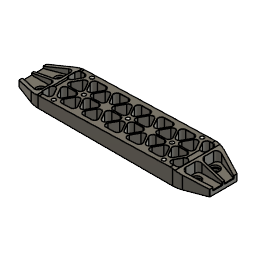
BUBBLED (Autodesk Fusion 360 design; units mm, degrees)
part number: 2026-08-30-08-59-27-515
Autodesk Fusion 360 part; units mm, degrees
note: some values were not read from the file. Chosen so that the rebuilt part matches the saved one: which face or edge a step refers to; how an offset face is resized.
sketch "Sketch1" plane through (0, 0, 0) normal (0, 1, 0) x (1, 0, 0)
  line L0 (30.0059, 0) -> (173.1941, 0)
  line L1 (203.2, -9.789) -> (203.2, -38.471)
  line L2 (173.1941, -48.26) -> (30.0059, -48.26)
  line L3 (0, -38.471) -> (0, -9.789)
  line L4 (0.2472, -9.4323) -> (21.0874, -1.6172)
  line L5 (21.0874, -46.6428) -> (0.2472, -38.8277)
  line L6 (182.1126, -1.6172) -> (202.9528, -9.4323)
  line L7 (202.9528, -38.8277) -> (182.1126, -46.6428)
  arc A0 (21.0874, -46.6428) -> (30.0059, -48.26) centre (30.0059, -22.86) ccw
  arc A1 (173.1941, -48.26) -> (182.1126, -46.6428) centre (173.1941, -22.86) ccw
  arc A2 (182.1126, -1.6172) -> (173.1941, 0) centre (173.1941, -25.4) ccw
  arc A3 (30.0059, 0) -> (21.0874, -1.6172) centre (30.0059, -25.4) ccw
  arc A4 (0.2472, -9.4323) -> (0, -9.789) centre (0.381, -9.789) ccw
  arc A5 (0, -38.471) -> (0.2472, -38.8277) centre (0.381, -38.471) ccw
  arc A6 (202.9528, -38.8277) -> (203.2, -38.471) centre (202.819, -38.471) ccw
  arc A7 (203.2, -9.789) -> (202.9528, -9.4323) centre (202.819, -9.789) ccw
  point P0 (0, -9.525)
  point P1 (25.4, 0)
  dimension "d5" = 25.4
  dimension "d6" = 9.525
  dimension "d13" = 25.4
  dimension "d14" = 0.381
  constraint horizontal L0
  constraint vertical L1
  constraint horizontal L2
  constraint vertical L3
  constraint tangent L5 A0
  constraint tangent L2 A0
  constraint tangent L7 A1
  constraint tangent L2 A1
  constraint equal A0 A1
  constraint tangent L6 A2
  constraint tangent L0 A2
  constraint equal A0 A2
  constraint coincident P1 L4
  constraint coincident L0 P1
  constraint tangent L4 A3
  constraint tangent L0 A3
  constraint equal A0 A3
  constraint coincident P0 L4
  constraint coincident L3 P0
  constraint tangent L4 A4
  constraint tangent L3 A4
  constraint tangent L5 A5
  constraint tangent L3 A5
  constraint equal A4 A5
  constraint tangent L7 A6
  constraint tangent L1 A6
  constraint equal A4 A6
  constraint tangent L6 A7
  constraint tangent L1 A7
  constraint equal A4 A7
  measures "d5" distance of origin P1
  measures "d6" distance of origin P0
  measures "d13" radius of A0
  measures "d14" radius of A4
extrude "Extrude1" add sketch "Sketch1" along normal blind 22.2504
sketch "Sketch2" plane through (0, 0, 0) normal (0, -1, 0) x (1, 0, 0)
  arc A0 (203.2, 38.471) -> (202.9528, 38.8277) centre (202.819, 38.471) ccw
  line L0 (202.9528, 38.8277) -> (182.1126, 46.6428)
  arc A1 (182.1126, 46.6428) -> (173.1941, 48.26) centre (173.1941, 22.86) ccw
  line L1 (173.1941, 48.26) -> (30.0059, 48.26)
  arc A2 (30.0059, 48.26) -> (21.0874, 46.6428) centre (30.0059, 22.86) ccw
  line L2 (21.0874, 46.6428) -> (0.2472, 38.8277)
  arc A3 (0.2472, 38.8277) -> (0, 38.471) centre (0.381, 38.471) ccw
  line L3 (0, 38.471) -> (0, 9.789)
  arc A4 (0, 9.789) -> (0.2472, 9.4323) centre (0.381, 9.789) ccw
  line L4 (0.2472, 9.4323) -> (21.0874, 1.6172)
  arc A5 (21.0874, 1.6172) -> (30.0059, 0) centre (30.0059, 25.4) ccw
  line L5 (30.0059, 0) -> (173.1941, 0)
  arc A6 (173.1941, 0) -> (182.1126, 1.6172) centre (173.1941, 25.4) ccw
  line L6 (182.1126, 1.6172) -> (202.9528, 9.4323)
  arc A7 (202.9528, 9.4323) -> (203.2, 9.789) centre (202.819, 9.789) ccw
  line L7 (203.2, 9.789) -> (203.2, 38.471)
  circle A8 centre (101.6, 24.13) radius 3.4925
  circle A9 centre (54.6608, 24.13) radius 3.4925
  circle A10 centre (148.5392, 24.13) radius 3.4925
  dimension "d17" = 6.985
  dimension "d18" = 24.13
  dimension "d19" = 101.6
  dimension "d22" = 46.9392
  dimension "d23" = 0
  measures "d17" diameter of A8
  measures "d18" distance of L1 A8.centre
  measures "d19" distance of L3 A8.centre
extrude "Extrude2" cut sketch "Sketch2" against normal blind 5.08
sketch "Sketch3" plane through (0, 22.2504, 0) normal (0, 1, 0) x (-1, 0, 0)
  arc A0 (-202.9528, 38.8277) -> (-203.2, 38.471) centre (-202.819, 38.471) ccw
  line L0 (-203.2, 38.471) -> (-203.2, 9.789)
  arc A1 (-203.2, 9.789) -> (-202.9528, 9.4323) centre (-202.819, 9.789) ccw
  line L1 (-202.9528, 9.4323) -> (-182.1126, 1.6172)
  arc A2 (-182.1126, 1.6172) -> (-173.1941, 0) centre (-173.1941, 25.4) ccw
  line L2 (-173.1941, 0) -> (-30.0059, 0)
  arc A3 (-30.0059, 0) -> (-21.0874, 1.6172) centre (-30.0059, 25.4) ccw
  line L3 (-21.0874, 1.6172) -> (-0.2472, 9.4323)
  arc A4 (-0.2472, 9.4323) -> (0, 9.789) centre (-0.381, 9.789) ccw
  line L4 (0, 9.789) -> (0, 38.471)
  arc A5 (0, 38.471) -> (-0.2472, 38.8277) centre (-0.381, 38.471) ccw
  line L5 (-0.2472, 38.8277) -> (-21.0874, 46.6428)
  arc A6 (-21.0874, 46.6428) -> (-30.0059, 48.26) centre (-30.0059, 22.86) ccw
  line L6 (-30.0059, 48.26) -> (-173.1941, 48.26)
  arc A7 (-173.1941, 48.26) -> (-182.1126, 46.6428) centre (-173.1941, 22.86) ccw
  line L7 (-182.1126, 46.6428) -> (-202.9528, 38.8277)
  line L8 (-101.6, -25.4) -> (-101.6, 76.2) construction
  point P0 (-101.6, 24.13)
  point P1 (-42.9514, 3.81)
  point P2 (-42.9514, 44.45)
  point P3 (-54.6608, 24.13)
  point P4 (-148.5392, 24.13)
  point P5 (-160.2486, 3.81)
  point P6 (-160.2486, 44.45)
  dimension "d26" = 24.13
  dimension "d27" = 101.6
  dimension "d28" = 3.81
  dimension "d29" = 42.9514
  dimension "d30" = 42.9514
  dimension "d31" = 44.45
  dimension "d32" = 24.13
  dimension "d33" = 54.6608
  constraint vertical L8
  constraint symmetric L8 P1 P5
  constraint symmetric L8 P2 P6
  constraint symmetric L8 P3 P4
  measures "d26" distance of L2 P0
  measures "d27" distance of L4 P0
  measures "d28" distance of L2 P1
  measures "d29" distance of L4 P1
  measures "d30" distance of L4 P2
  measures "d31" distance of L2 P2
  measures "d32" distance of L2 P3
  measures "d33" distance of L4 P3
sketch "Sketch4" plane through (0, 22.2504, 0) normal (0, 1, 0) x (-1, 0, 0)
  line L0 (-27.94, 7.0358) -> (-27.94, 13.7682)
  line L1 (-33.9594, 15.3811) -> (-37.8464, 8.6487)
  line L2 (-35.0528, 3.81) -> (-31.1658, 3.81)
  line L3 (-173.1941, 0) -> (-30.0059, 0)
  line L4 (0, 9.789) -> (0, 38.471)
  arc A0 (-31.1658, 3.81) -> (-27.94, 7.0358) centre (-31.1658, 7.0358) ccw
  arc A1 (-37.8464, 8.6487) -> (-35.0528, 3.81) centre (-35.0528, 7.0358) ccw
  arc A2 (-27.94, 13.7682) -> (-33.9594, 15.3811) centre (-31.1658, 13.7682) ccw
  line L5 (-101.6, -25.4) -> (-101.6, 76.2) construction
  line L6 (-169.2406, 15.3811) -> (-165.3536, 8.6487)
  arc A3 (-169.2406, 15.3811) -> (-175.26, 13.7682) centre (-172.0342, 13.7682) ccw
  arc A4 (-168.1473, 3.81) -> (-165.3536, 8.6487) centre (-168.1473, 7.0358) ccw
  line L7 (-168.1473, 3.81) -> (-172.0342, 3.81)
  arc A5 (-175.26, 7.0358) -> (-172.0342, 3.81) centre (-172.0342, 7.0358) ccw
  line L8 (-175.26, 7.0358) -> (-175.26, 13.7682)
  dimension "d34" = 3.81
  dimension "d35" = 27.94
  dimension "d36" = 60
  dimension "d37" = 3.2258
  dimension "d102" = 101.6
  constraint vertical L0
  constraint perpendicular L0 L2
  constraint tangent L0 A0
  constraint tangent L2 A0
  constraint tangent L1 A1
  constraint tangent L2 A1
  constraint equal A0 A1
  constraint tangent L0 A2
  constraint tangent L1 A2
  constraint equal A0 A2
  constraint perpendicular L3 L5
  constraint symmetric L0.start L5 A5.start
  constraint symmetric L2.end L5 L7.end
  constraint symmetric A0 L5 A5
  constraint symmetric L1.end L5 L6.end
  constraint symmetric L2.start L5 A4.start
  constraint symmetric A1 L5 A4
  constraint symmetric L0.end L5 A3.end
  constraint symmetric L1.start L5 L6.start
  constraint symmetric A2 L5 A3
  measures "d34" distance of L2 L3
  measures "d35" distance of L0 L4
  measures "d36" angle of L1 L2
  measures "d37" radius of A0
  measures "d102" distance of origin L5
sketch "Sketch5" plane through (0, 22.2504, 0) normal (0, 1, 0) x (-1, 0, 0)
  line L0 (-42.929, 3.81) -> (-31.1973, 24.13) construction
  line L1 (-31.1973, 24.13) -> (-42.929, 44.45) construction
  line L2 (-42.929, 44.45) -> (-66.3926, 44.45) construction
  line L3 (-66.3926, 44.45) -> (-78.1243, 24.13) construction
  line L4 (-78.1243, 24.13) -> (-66.3926, 3.81) construction
  line L5 (-66.3926, 3.81) -> (-42.929, 3.81) construction
  line L6 (-54.6608, 24.13) -> (-78.1243, 24.13) construction
  line L7 (-66.0614, 3.81) -> (-66.3926, 44.45) construction
  line L8 (-63.3332, 10.1409) -> (-58.7834, 18.0213)
  line L9 (-61.577, 22.86) -> (-70.6783, 22.86)
  line L10 (-73.4716, 18.0208) -> (-68.9202, 10.1404)
  line L11 (-173.1941, 0) -> (-30.0059, 0) construction
  arc A0 (-68.9202, 10.1404) -> (-63.3332, 10.1409) centre (-66.1268, 11.7538) ccw
  arc A1 (-58.7834, 18.0213) -> (-61.577, 22.86) centre (-61.577, 19.6342) ccw
  arc A2 (-70.6783, 22.86) -> (-73.4716, 18.0208) centre (-70.6783, 19.6342) ccw
  line L12 (-58.7755, 4.7847) -> (-49.6751, 4.7862)
  arc A3 (-61.5697, 9.6234) -> (-58.7755, 4.7847) centre (-58.7761, 8.0105) ccw
  line L13 (-57.0191, 17.5054) -> (-61.5697, 9.6234)
  arc A4 (-49.6751, 4.7862) -> (-46.882, 9.6249) centre (-49.6757, 8.012) ccw
  arc A5 (-51.4318, 17.5054) -> (-57.0191, 17.5054) centre (-54.2254, 15.8925) ccw
  line L14 (-46.882, 9.6249) -> (-51.4318, 17.5054)
  line L15 (-39.9647, 10.8939) -> (-35.4158, 18.7758)
  arc A6 (-45.5522, 10.8934) -> (-39.9647, 10.8939) centre (-42.7586, 12.5063) ccw
  line L16 (-50.1028, 18.7754) -> (-45.5522, 10.8934)
  arc A7 (-35.4158, 18.7758) -> (-38.2097, 23.6141) centre (-38.2097, 20.3883) ccw
  arc A8 (-47.3092, 23.6141) -> (-50.1028, 18.7754) centre (-47.3092, 20.3883) ccw
  line L17 (-38.2097, 23.6141) -> (-47.3092, 23.6141)
  line L18 (-35.85, 30.2392) -> (-40.4014, 38.1196)
  arc A9 (-38.6433, 25.4) -> (-35.85, 30.2392) centre (-38.6433, 28.6258) ccw
  line L19 (-47.7446, 25.4) -> (-38.6433, 25.4)
  arc A10 (-40.4014, 38.1196) -> (-45.9884, 38.1191) centre (-43.1948, 36.5062) ccw
  arc A11 (-50.5382, 30.2387) -> (-47.7446, 25.4) centre (-47.7446, 28.6258) ccw
  line L20 (-45.9884, 38.1191) -> (-50.5382, 30.2387)
  line L21 (-50.5461, 43.4753) -> (-59.6465, 43.4738)
  arc A12 (-47.7519, 38.6366) -> (-50.5461, 43.4753) centre (-50.5455, 40.2495) ccw
  line L22 (-52.3025, 30.7546) -> (-47.7519, 38.6366)
  arc A13 (-59.6465, 43.4738) -> (-62.4396, 38.6351) centre (-59.6459, 40.248) ccw
  arc A14 (-57.8898, 30.7546) -> (-52.3025, 30.7546) centre (-55.0962, 32.3675) ccw
  line L23 (-62.4396, 38.6351) -> (-57.8898, 30.7546)
  line L24 (-69.3569, 37.3661) -> (-73.9058, 29.4842)
  arc A15 (-63.7694, 37.3666) -> (-69.3569, 37.3661) centre (-66.563, 35.7537) ccw
  line L25 (-59.2188, 29.4846) -> (-63.7694, 37.3666)
  arc A16 (-73.9058, 29.4842) -> (-71.1119, 24.6459) centre (-71.1119, 27.8717) ccw
  arc A17 (-62.0124, 24.6459) -> (-59.2188, 29.4846) centre (-62.0124, 27.8717) ccw
  line L26 (-71.1119, 24.6459) -> (-62.0124, 24.6459)
  point P0 (-54.6608, 24.13)
  point P1 (-54.6608, 24.13)
  dimension "d38" = 20.32
  dimension "d39" = 1.27
  dimension "d40" = 59.991
  dimension "d41" = 3.2258
  dimension "d43" = 360
  constraint coincident P0 L6.start
  constraint coincident L5 L7.start
  constraint horizontal L6
  constraint parallel L6 L9
  constraint tangent L8 A0
  constraint tangent L10 A0
  constraint tangent L8 A1
  constraint tangent L9 A1
  constraint equal A0 A1
  constraint tangent L9 A2
  constraint tangent L10 A2
  constraint equal A0 A2
  measures "d38" distance of P1 L5
  measures "d39" distance of L6 L9
  measures "d40" angle of L10 L11
  measures "d41" radius of A0
sketch "Sketch6" plane through (0, 22.2504, 0) normal (0, 1, 0) x (-1, 0, 0)
  line L0 (-57.0191, 17.5054) -> (-61.5697, 9.6234) construction
  arc A0 (-61.5697, 9.6234) -> (-58.7755, 4.7847) centre (-58.7761, 8.0105) ccw construction
  line L1 (-58.7755, 4.7847) -> (-49.6751, 4.7862) construction
  arc A1 (-49.6751, 4.7862) -> (-46.882, 9.6249) centre (-49.6757, 8.012) ccw construction
  line L2 (-46.882, 9.6249) -> (-51.4318, 17.5054) construction
  arc A2 (-51.4318, 17.5054) -> (-57.0191, 17.5054) centre (-54.2254, 15.8925) ccw construction
  line L3 (-66.0614, 3.81) -> (-66.3926, 44.45)
  arc A3 (-73.3622, 4.6659) -> (-70.6472, 9.5495) centre (-73.4142, 7.8913) ccw
  line L4 (-73.3622, 4.6659) -> (-82.4614, 4.5191)
  arc A4 (-85.333, 9.3116) -> (-82.4614, 4.5191) centre (-82.5134, 7.7444) ccw
  line L5 (-85.333, 9.3116) -> (-80.9122, 17.2651)
  arc A5 (-75.3257, 17.3562) -> (-80.9122, 17.2651) centre (-78.0927, 15.698) ccw
  line L6 (-75.3257, 17.3562) -> (-70.6472, 9.5495)
  line L7 (-101.6, -25.4) -> (-101.6, 72.1933) construction
  arc A6 (-120.7386, 4.5191) -> (-117.867, 9.3116) centre (-120.6866, 7.7444) ccw
  line L8 (-117.867, 9.3116) -> (-122.2878, 17.2651)
  line L9 (-127.8743, 17.3562) -> (-132.5528, 9.5495)
  arc A7 (-132.5528, 9.5495) -> (-129.8378, 4.6659) centre (-129.7858, 7.8913) ccw
  arc A8 (-122.2878, 17.2651) -> (-127.8743, 17.3562) centre (-125.1073, 15.698) ccw
  line L10 (-129.8378, 4.6659) -> (-120.7386, 4.5191)
  dimension "d95" = 101.6
  constraint symmetric L0.start L3 A5.start
  constraint symmetric L0.end L3 A3.end
  constraint symmetric A0.end L3 A3.start
  constraint symmetric A0 L3 A3
  constraint symmetric L1.end L3 L4.end
  constraint symmetric A1.end L3 A4.start
  constraint symmetric A1 L3 A4
  constraint symmetric L2.end L3 L5.end
  constraint symmetric A2 L3 A5
  constraint vertical L7
  constraint symmetric A3.end L7 L9.end
  constraint symmetric A3.start L7 A7.end
  constraint symmetric A3 L7 A7
  constraint symmetric L4.end L7 A6.start
  constraint symmetric A4.start L7 A6.end
  constraint symmetric A4 L7 A6
  constraint symmetric L5.end L7 L8.end
  constraint symmetric A5.start L7 L9.start
  constraint symmetric A5 L7 A8
  measures "d95" distance of origin L7
sketch "Sketch7" plane through (0, 22.2504, 0) normal (0, 1, 0) x (-1, 0, 0)
  line L0 (0, 9.789) -> (0, 38.471)
  line L1 (-173.1941, 0) -> (-30.0059, 0)
  line L2 (-101.6, -25.4) -> (-101.6, 76.2)
  point P0 (-18.923, 14.1732)
  point P1 (-18.923, 34.0868)
  point P2 (-184.277, 14.1732)
  point P3 (-184.277, 34.0868)
  dimension "d45" = 18.923
  dimension "d46" = 18.923
  dimension "d47" = 14.1732
  dimension "d48" = 34.0868
  constraint symmetric P0 L2 P2
  constraint symmetric P1 L2 P3
  measures "d45" distance of P0 L0
  measures "d46" distance of P1 L0
  measures "d47" distance of P0 L1
  measures "d48" distance of P1 L1
sketch "Sketch8" plane through (0, 22.2504, 0) normal (0, 1, 0) x (-1, 0, 0)
  line L0 (12.6994, 18.0851) -> (12.6994, 22.86)
  line L1 (12.6994, 22.86) -> (-21.59, 22.86)
  line L2 (-25.4, 19.05) -> (-25.4, 9.2956)
  line L3 (-20.2522, 5.7282) -> (12.6994, 18.0851)
  line L4 (-21.0874, 1.6172) -> (-0.2472, 9.4323)
  line L5 (0, 9.789) -> (0, 38.471)
  line L6 (-173.1941, 0) -> (-30.0059, 0)
  line L7 (12.7, 24.13) -> (-76.2, 24.13) construction
  arc A0 (-25.4, 9.2956) -> (-20.2522, 5.7282) centre (-21.59, 9.2956) ccw
  arc A1 (-21.59, 22.86) -> (-25.4, 19.05) centre (-21.59, 19.05) ccw
  line L8 (12.6994, 25.4) -> (-21.59, 25.4)
  arc A2 (-25.4, 29.21) -> (-21.59, 25.4) centre (-21.59, 29.21) ccw
  line L9 (-25.4, 29.21) -> (-25.4, 38.9644)
  arc A3 (-20.2522, 42.5318) -> (-25.4, 38.9644) centre (-21.59, 38.9644) ccw
  line L10 (-20.2522, 42.5318) -> (12.6994, 30.1749)
  line L11 (12.6994, 30.1749) -> (12.6994, 25.4)
  line L12 (-101.6, -25.4) -> (-101.6, 76.2) construction
  line L13 (-177.8, 19.05) -> (-177.8, 9.2956)
  arc A4 (-182.9478, 5.7282) -> (-177.8, 9.2956) centre (-181.61, 9.2956) ccw
  line L14 (-182.9478, 5.7282) -> (-215.8994, 18.0851)
  line L15 (-215.8994, 18.0851) -> (-215.8994, 22.86)
  line L16 (-215.8994, 22.86) -> (-181.61, 22.86)
  arc A5 (-177.8, 19.05) -> (-181.61, 22.86) centre (-181.61, 19.05) ccw
  arc A6 (-181.61, 25.4) -> (-177.8, 29.21) centre (-181.61, 29.21) ccw
  line L17 (-215.8994, 25.4) -> (-181.61, 25.4)
  line L18 (-177.8, 29.21) -> (-177.8, 38.9644)
  arc A7 (-177.8, 38.9644) -> (-182.9478, 42.5318) centre (-181.61, 38.9644) ccw
  line L19 (-182.9478, 42.5318) -> (-215.8994, 30.1749)
  line L20 (-215.8994, 30.1749) -> (-215.8994, 25.4)
  dimension "d50" = 3.556
  dimension "d51" = 25.4
  dimension "d52" = 22.86
  dimension "d53" = 3.81
  dimension "d54" = 24.13
  constraint vertical L0
  constraint perpendicular L0 L1
  constraint perpendicular L1 L2
  constraint parallel L3 L4
  constraint horizontal L7
  constraint tangent L2 A0
  constraint tangent L3 A0
  constraint tangent L1 A1
  constraint tangent L2 A1
  constraint equal A0 A1
  constraint symmetric L0.start L7 L10.end
  constraint symmetric L0.end L7 L8.start
  constraint symmetric L7 L2.end L9.end
  constraint symmetric L7 L3.start A3.start
  constraint symmetric L7 A0 A3
  constraint symmetric L7 L1.end L8.end
  constraint symmetric L7 L2.start A2.start
  constraint symmetric L7 A1 A2
  constraint symmetric L0.start L12 L14.end
  constraint symmetric L0.end L12 L15.end
  constraint symmetric L2.end L12 L13.end
  constraint symmetric L3.start L12 A4.start
  constraint symmetric A0 L12 A4
  constraint symmetric L1.end L12 L16.end
  constraint symmetric L2.start L12 L13.start
  constraint symmetric A1 L12 A5
  constraint symmetric L8.start L12 L17.start
  constraint symmetric L8.end L12 A6.start
  constraint symmetric A2.start L12 A6.end
  constraint symmetric A2 L12 A6
  constraint symmetric L9.end L12 L18.end
  constraint symmetric A3.start L12 A7.end
  constraint symmetric A3 L12 A7
  constraint symmetric L10.end L12 L19.end
  measures "d50" distance of L3 L4
  measures "d51" distance of L2 L5
  measures "d52" distance of L1 L6
  measures "d53" radius of A0
  measures "d54" distance of L6 L7
sketch "Sketch9" plane through (0, 0, 48.26) normal (0, 0, 1) x (1, 0, 0)
  line L0 (30.0059, 5.08) -> (173.1941, 5.08) construction
  line L1 (173.1941, 5.08) -> (173.1941, 22.2504)
  line L2 (173.1941, 22.2504) -> (30.0059, 22.2504)
  line L3 (30.0059, 22.2504) -> (30.0059, 5.08)
  line L4 (30.0059, 5.08) -> (173.1941, 5.08)
  line L5 (0, 5.08) -> (0, 11.4554)
  line L6 (30.0059, 5.08) -> (30.0059, 17.1704)
  line L7 (0, 11.4554) -> (30.0059, 17.1704)
  line L8 (30.0059, 22.2504) -> (0, 22.2504)
  line L9 (0, 22.2504) -> (0, 11.4554)
  line L10 (30.0059, 17.1704) -> (30.0059, 22.2504)
  line L11 (30.0059, 22.2504) -> (203.2, 22.2504)
  line L12 (203.2, 22.2504) -> (203.2, 12.0904)
  line L13 (30.0059, 17.1704) -> (173.1941, 21.4376)
  line L14 (203.2, 12.0904) -> (173.1941, 21.4376)
  point P0 (0, 5.08)
  dimension "d57" = 10.795
  dimension "d58" = 5.08
  dimension "d61" = 10.16
  dimension "d62" = 21.4376
  constraint coincident P0 L5.start
  constraint vertical L5
  constraint coincident L0.start L3.end
  constraint coincident L3 L6.end
  constraint coincident L2.end L3.start
  constraint perpendicular L3 L8
  constraint perpendicular L8 L9
  constraint perpendicular L3 L11
  constraint perpendicular L11 L12
  constraint coincident L1 L13.end
  measures "d57" distance of L2 L5.end
  measures "d58" distance of L2 L6.end
  measures "d61" distance of L11.end L12.end
  measures "d62" vertical distance of origin L13.end
extrude "Extrude3" cut sketch "Sketch9" against normal blind 76.2 contours L1 L2 L3 L10 L11 L13 | L1 L11 L12 L14 | L3 L7 L8 L9 L10
fillet "Fillet1" radius 15.24 2 edges at (173.1941, 21.4376, 24.13) (30.0059, 17.1704, 24.13)
hole "Hole1" at (42.9514, 22.2504, 3.81) at (54.6608, 22.2504, 24.13) at (42.9514, 22.2504, 44.45) at (160.2486, 22.2504, 44.45) at (148.5392, 22.2504, 24.13) at (160.2486, 22.2504, 3.81) at (101.6, 22.2504, 24.13) direction (0, -1, 0) diameter 3.9688 depth 22.8203 tip angle 118
thread "Thread1" "ANSI Unified Screw Threads 0.19(#10) 10-32 UNF 10-32 UNF 2B" major diameter 4.826 minor diameter 4.064 pitch 0.7937 angle 60 resizes the face on face at (44.846, 9.2575, 4.4001) on face at (162.1424, 10.4227, 4.4025) on face at (56.6452, 5.9881, 24.1326) on face at (44.846, 9.2575, 45.0401) on face at (162.1424, 10.4227, 45.0425) on face at (103.5603, 6.4541, 24.4383) on face at (150.4364, 6.9198, 24.7116)
extrude "Extrude4" cut sketch "Sketch8" against normal blind 12.7 contours L1 L2 L3 L5 A0 A1 | L5 L8 A2 L9 A3 L10 | L13 A4 L14 L15 L16 A5 | A6 L17 L18 A7 L19 L20
fillet "Fillet2" radius 0.381 12 edges at (203.2, 10.8204, 13.3228) (203.2, 9.5504, 18.0914) (203.2, 10.8204, 22.86) (203.2, 10.8204, 25.4) (203.2, 9.5504, 30.1686) (203.2, 10.8204, 34.9372) (0, 10.5029, 13.3228) (0, 9.5504, 18.0914) (0, 10.5029, 22.86) (0, 10.5029, 25.4) (0, 9.5504, 30.1686) (0, 10.5029, 34.9372)
sketch "Sketch10" plane through (0, 9.5504, 0) normal (0, 1, 0) x (-1, 0, 0)
  line L0 (-0.381, 25.4) -> (-0.381, 35.106)
  arc A0 (-0.5148, 35.1302) -> (-0.381, 35.106) centre (-0.381, 35.487) ccw
  line L1 (-0.5148, 35.1302) -> (-20.2522, 42.5318)
  arc A1 (-20.2522, 42.5318) -> (-25.4, 38.9644) centre (-21.59, 38.9644) ccw
  line L2 (-25.4, 38.9644) -> (-25.4, 29.21)
  arc A2 (-25.4, 29.21) -> (-21.59, 25.4) centre (-21.59, 29.21) ccw
  line L3 (-21.59, 25.4) -> (-0.381, 25.4)
  line L4 (0, 9.789) -> (0, 38.471)
  point P0 (-184.277, 34.0868)
  point P1 (-184.277, 14.1732)
  point P2 (-18.923, 14.1732)
  point P3 (-18.923, 34.0868)
  dimension "d86" = 18.8516
hole "Hole3" at (18.923, 9.5504, 34.0868) at (18.923, 9.5504, 14.1732) at (184.277, 9.5504, 14.1732) at (184.277, 9.5504, 34.0868) direction (0, -1, 0) diameter 6.604 depth 5.08 tip angle 118 counterbore diameter 9.652 counterbore depth 2.032
extrude "Extrude5" cut sketch "Sketch5" against normal blind 20.2406
pattern_linear "R-Pattern1" count 3 spacing 47.0297 along (0.999556, 0.029788, 0) of "Extrude5"
extrude "Extrude6" cut sketch "Sketch6" against normal blind 20.2406
ref_plane "WorkPlane1" through (0, 0, 24.13) normal (0, 0, 1) x (1, 0, 0)
mirror "Mirror1" about plane through (0, 0, 24.13) normal (0, 0, 1) of "Extrude6"
extrude "Extrude7" cut sketch "Sketch4" against normal blind 20.2406
mirror "Mirror2" about plane through (0, 0, 24.13) normal (0, 0, 1) of "Extrude7"
chamfer "Chamfer1" distance 0.127 angle 45 324 edges at (171.3392, 21.3664, 44.45) (174.4878, 20.9865, 43.3184) (175.26, 20.7889, 37.858) (174.0492, 21.0798, 31.9727) (174.0492, 21.0798, 16.2873) (175.26, 20.7889, 10.402) (174.4878, 20.9865, 4.9416) (171.3392, 21.3664, 3.81) (33.1093, 5.08, 3.81) (28.8848, 5.08, 4.7548) (37.8464, 5.08, 5.4229) (27.94, 5.08, 10.402) (35.9029, 5.08, 12.0149) (30.3309, 5.08, 16.8841) (59.2944, 5.08, 13.5644) (61.5696, 5.08, 6.3974) (54.2254, 5.08, 19.1183) (54.2253, 5.08, 4.7855) (49.1569, 5.08, 13.5651) (46.8819, 5.08, 6.3994) (85.2805, 5.08, 6.0865) (83.1226, 5.08, 13.2884) (77.9118, 5.08, 4.5925) (78.1452, 5.08, 18.9233) (70.5948, 5.08, 6.3239) (72.9865, 5.08, 13.4528) (106.3032, 5.08, 13.5644) (108.5784, 5.08, 6.3974) (101.2343, 5.08, 19.1183) (101.2342, 5.08, 4.7855) (96.1658, 5.08, 13.5651) (93.8907, 5.08, 6.3994) (47.8275, 5.08, 14.8344) (42.7583, 5.08, 9.2805) (50.1028, 5.08, 22.0012) (37.6902, 5.08, 14.8349) (42.7594, 5.08, 23.6141) (35.4162, 5.08, 22.0014) (71.1959, 5.08, 14.0806) (66.1265, 5.08, 8.528) (73.472, 5.08, 21.2469) (61.0583, 5.08, 14.0811) (66.1277, 5.08, 22.86) (58.7834, 5.08, 21.2471) (94.8363, 5.08, 14.8344) (89.7671, 5.08, 9.2805) (97.1116, 5.08, 22.0012) (84.6991, 5.08, 14.8349) (89.7683, 5.08, 23.6141) (82.425, 5.08, 22.0014) (125.2882, 5.08, 4.5925) (117.9195, 5.08, 6.0865) (132.6052, 5.08, 6.3239) (120.0774, 5.08, 13.2884) (130.2135, 5.08, 13.4528) (125.0548, 5.08, 18.9233) (153.312, 5.08, 13.5644) (155.5872, 5.08, 6.3974) (148.2431, 5.08, 19.1183) (148.243, 5.08, 4.7855) (143.1746, 5.08, 13.5651) (140.8996, 5.08, 6.3994) (165.3536, 5.08, 5.4229) (170.0907, 5.08, 3.81) (167.2971, 5.08, 12.0149) (174.3152, 5.08, 4.7548) (172.8691, 5.08, 16.8841) (175.26, 5.08, 10.402) (118.2047, 5.08, 14.0806) (113.1354, 5.08, 8.528) (120.4809, 5.08, 21.2469) (108.0671, 5.08, 14.0811) (113.1365, 5.08, 22.86) (105.7922, 5.08, 21.2471) (141.8452, 5.08, 14.8344) (136.776, 5.08, 9.2805) (144.1205, 5.08, 22.0012) (131.7079, 5.08, 14.8349) (136.7771, 5.08, 23.6141) (129.4338, 5.08, 22.0014) (165.2135, 5.08, 14.0806) (160.1442, 5.08, 8.528) (167.4897, 5.08, 21.2469) (155.0759, 5.08, 14.0811) (160.1453, 5.08, 22.86) (152.801, 5.08, 21.2471) (43.1939, 5.08, 25.4) (35.8496, 5.08, 27.0131) (50.5382, 5.08, 27.0129) (38.1257, 5.08, 34.1794) (48.2633, 5.08, 34.1789) (43.1951, 5.08, 39.732) (61.4941, 5.08, 33.4256) (66.5633, 5.08, 38.9795) (59.2188, 5.08, 26.2588) (71.6314, 5.08, 33.4251) (66.5622, 5.08, 24.6459) (73.9054, 5.08, 26.2586) (90.2028, 5.08, 25.4) (82.8584, 5.08, 27.0131) (97.547, 5.08, 27.0129) (85.1345, 5.08, 34.1794) (95.2721, 5.08, 34.1789) (90.2039, 5.08, 39.732) (27.94, 5.08, 37.858) (30.3309, 5.08, 31.3759) (35.9029, 5.08, 36.2451) (37.8464, 5.08, 42.8371) (33.1093, 5.08, 44.45) (28.8848, 5.08, 43.5052) (50.0272, 5.08, 34.6956) (47.752, 5.08, 41.8626) (55.0962, 5.08, 29.1417) (55.0963, 5.08, 43.4745) (60.1647, 5.08, 34.6949) (62.4397, 5.08, 41.8606) (77.9118, 5.08, 43.6675) (85.2805, 5.08, 42.1735) (70.5948, 5.08, 41.9361) (83.1226, 5.08, 34.9716) (72.9865, 5.08, 34.8072) (78.1452, 5.08, 29.3367) (108.5029, 5.08, 33.4256) (113.5721, 5.08, 38.9795) (106.2276, 5.08, 26.2588) (118.6402, 5.08, 33.4251) (113.571, 5.08, 24.6459) (120.9142, 5.08, 26.2586) (137.2116, 5.08, 25.4) (129.8672, 5.08, 27.0131) (144.5558, 5.08, 27.0129) (132.1433, 5.08, 34.1794) (142.2809, 5.08, 34.1789) (137.2127, 5.08, 39.732) (155.5117, 5.08, 33.4256) (160.5809, 5.08, 38.9795) (153.2364, 5.08, 26.2588) (165.649, 5.08, 33.4251) (160.5798, 5.08, 24.6459) (167.9231, 5.08, 26.2586) (97.036, 5.08, 34.6956) (94.7609, 5.08, 41.8626) (102.105, 5.08, 29.1417) (102.1051, 5.08, 43.4745) (107.1735, 5.08, 34.6949) (109.4485, 5.08, 41.8606) (117.9195, 5.08, 42.1735) (120.0774, 5.08, 34.9716) (125.2882, 5.08, 43.6675) (125.0548, 5.08, 29.3367) (132.6052, 5.08, 41.9361) (130.2135, 5.08, 34.8072) (144.0449, 5.08, 34.6956) (141.7697, 5.08, 41.8626) (149.1138, 5.08, 29.1417) (149.1139, 5.08, 43.4745) (154.1823, 5.08, 34.6949) (156.4573, 5.08, 41.8606) (167.2971, 5.08, 36.2451) (172.8691, 5.08, 31.3759) (175.26, 5.08, 37.858) (174.3152, 5.08, 43.5052) (170.0907, 5.08, 44.45) (165.3536, 5.08, 42.8371) (169.3954, 21.3244, 44.45) (165.3536, 21.2039, 42.8371) (167.2971, 21.2619, 36.2451) (169.8438, 21.3378, 32.1237) (169.8438, 21.3378, 16.1363) (167.2971, 21.2619, 12.0149) (165.3536, 21.2039, 5.4229) (169.3954, 21.3244, 3.81) (33.1339, 17.2636, 3.81) (37.8464, 17.4041, 5.4229) (35.9029, 17.3461, 12.0149) (32.8, 17.2537, 16.5494) (32.8, 17.2537, 31.7106) (35.9029, 17.3461, 36.2451) (37.8464, 17.4041, 42.8371) (33.1339, 17.2636, 44.45) (61.5696, 18.111, 6.3974) (54.2253, 17.8922, 4.7855) (59.2944, 18.0432, 13.5644) (46.8819, 17.6733, 6.3994) (54.2254, 17.8922, 19.1183) (49.1569, 17.7411, 13.5651) (85.2805, 18.8177, 6.0865) (77.9118, 18.5981, 4.5925) (83.1226, 18.7533, 13.2884) (70.5948, 18.38, 6.3239) (78.1452, 18.605, 18.9233) (72.9865, 18.4513, 13.4528) (108.5784, 19.512, 6.3974) (101.2342, 19.2931, 4.7855) (106.3032, 19.4442, 13.5644) (93.8907, 19.0743, 6.3994) (101.2343, 19.2931, 19.1183) (96.1658, 19.1421, 13.5651) (42.7583, 17.5504, 9.2805) (37.6902, 17.3994, 14.8349) (47.8275, 17.7015, 14.8344) (35.4162, 17.3316, 22.0014) (50.1028, 17.7693, 22.0012) (42.7594, 17.5505, 23.6141) (66.1265, 18.2468, 8.528) (61.0583, 18.0958, 14.0811) (71.1959, 18.3979, 14.0806) (58.7834, 18.028, 21.2471) (73.472, 18.4657, 21.2469) (66.1277, 18.2469, 22.86) (89.7671, 18.9514, 9.2805) (84.6991, 18.8003, 14.8349) (94.8363, 19.1024, 14.8344) (82.425, 18.7326, 22.0014) (97.1116, 19.1702, 22.0012) (89.7683, 18.9514, 23.6141) (125.2882, 20.0099, 4.5925) (117.9195, 19.7903, 6.0865) (132.6052, 20.228, 6.3239) (120.0774, 19.8547, 13.2884) (130.2135, 20.1567, 13.4528) (125.0548, 20.003, 18.9233) (155.5872, 20.9129, 6.3974) (148.243, 20.694, 4.7855) (153.312, 20.8451, 13.5644) (140.8996, 20.4752, 6.3994) (148.2431, 20.694, 19.1183) (143.1746, 20.543, 13.5651) (113.1354, 19.6478, 8.528) (108.0671, 19.4967, 14.0811) (118.2047, 19.7988, 14.0806) (105.7922, 19.4289, 21.2471) (120.4809, 19.8667, 21.2469) (113.1365, 19.6478, 22.86) (136.776, 20.3523, 9.2805) (131.7079, 20.2013, 14.8349) (141.8452, 20.5034, 14.8344) (129.4338, 20.1335, 22.0014) (144.1205, 20.5712, 22.0012) (136.7771, 20.3523, 23.6141) (160.1442, 21.0487, 8.528) (155.0759, 20.8977, 14.0811) (165.2135, 21.1998, 14.0806) (152.801, 20.8299, 21.2471) (167.4897, 21.2676, 21.2469) (160.1453, 21.0487, 22.86) (35.8496, 17.3445, 27.0131) (38.1257, 17.4124, 34.1794) (43.1939, 17.5634, 25.4) (43.1951, 17.5635, 39.732) (50.5382, 17.7823, 27.0129) (48.2633, 17.7145, 34.1789) (66.5633, 18.2599, 38.9795) (71.6314, 18.4109, 33.4251) (61.4941, 18.1088, 33.4256) (73.9054, 18.4787, 26.2586) (59.2188, 18.041, 26.2588) (66.5622, 18.2598, 24.6459) (82.8584, 18.7455, 27.0131) (85.1345, 18.8133, 34.1794) (90.2028, 18.9643, 25.4) (90.2039, 18.9644, 39.732) (97.547, 19.1832, 27.0129) (95.2721, 19.1154, 34.1789) (47.752, 17.6993, 41.8626) (55.0963, 17.9181, 43.4745) (50.0272, 17.7671, 34.6956) (62.4397, 18.137, 41.8606) (55.0962, 17.9181, 29.1417) (60.1647, 18.0692, 34.6949) (77.9118, 18.5981, 43.6675) (85.2805, 18.8177, 42.1735) (70.5948, 18.38, 41.9361) (83.1226, 18.7533, 34.9716) (72.9865, 18.4513, 34.8072) (78.1452, 18.605, 29.3367) (113.5721, 19.6608, 38.9795) (118.6402, 19.8118, 33.4251) (108.5029, 19.5097, 33.4256) (120.9142, 19.8796, 26.2586) (106.2276, 19.4419, 26.2588) (113.571, 19.6608, 24.6459) (129.8672, 20.1464, 27.0131) (132.1433, 20.2142, 34.1794) (137.2116, 20.3653, 25.4) (137.2127, 20.3653, 39.732) (144.5558, 20.5841, 27.0129) (142.2809, 20.5163, 34.1789) (160.5809, 21.0617, 38.9795) (165.649, 21.2127, 33.4251) (155.5117, 20.9106, 33.4256) (167.9231, 21.2805, 26.2586) (153.2364, 20.8428, 26.2588) (160.5798, 21.0617, 24.6459) (94.7609, 19.1002, 41.8626) (102.1051, 19.3191, 43.4745) (97.036, 19.168, 34.6956) (109.4485, 19.5379, 41.8606) (102.105, 19.319, 29.1417) (107.1735, 19.4701, 34.6949) (117.9195, 19.7903, 42.1735) (125.2882, 20.0099, 43.6675) (120.0774, 19.8547, 34.9716) (132.6052, 20.228, 41.9361) (125.0548, 20.003, 29.3367) (130.2135, 20.1567, 34.8072) (141.7697, 20.5011, 41.8626) (149.1139, 20.72, 43.4745) (144.0449, 20.5689, 34.6956) (156.4573, 20.9388, 41.8606) (149.1138, 20.72, 29.1417) (154.1823, 20.871, 34.6949) (31.1904, 17.2057, 3.81) (29.8196, 17.1006, 4.1043) (28.1674, 16.8202, 5.8461) (27.94, 16.7769, 10.402) (28.1674, 16.8202, 14.9579) (29.8363, 17.1026, 16.7073) (27.94, 16.7769, 37.858) (28.1674, 16.8202, 33.3021) (29.8363, 17.1026, 31.5527) (31.1904, 17.2057, 44.45) (29.8196, 17.1006, 44.1557) (28.1674, 16.8202, 42.4139)
equation "d23 = 0'-0\""
equation "d63 = -0'-3\""
equation "d67 = 0'- 115/128\""
equation "d68 = 0'- 5/32\""
equation "d70 = 0'-0\""
equation "d71 = 0'- 1/2\""
equation "d86 = 0'- 95/128\""
equation "d87 = -0'- 51/64\""
equation "d91 = -0'-3 45/64\""
equation "d92 = 0'-0\""
equation "d93 = -0'- 51/64\""
equation "d95 = 0'-4\""
equation "d97 = 0'-0\""
equation "d99 = 0'- 1/128\""
equation "d100 = -0'- 51/64\""
equation "d102 = 0'-4\""
equation "d104 = 0'- 1/128\""
